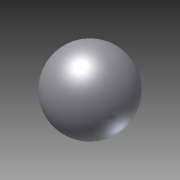
# Autodesk Inventor part: AtwoodsBall
Saved by Autodesk Inventor 2012 SP2 (Build 160219200, 219)
## iProperties
Created: 2013-07-18
Part Number: AtwoodsBall
Material: Default
Document SubType Name: Modeling
Designer: 1
Density: 1 g/cm^3
Author: 1
Autodesk Inventor part; units mm, degrees
ref_plane "YZ Plane" through (0, 0, 0) normal (1, 0, 0) x (0, 1, 0)
ref_plane "XZ Plane" through (0, 0, 0) normal (0, 1, 0) x (-1, 0, 0)
ref_plane "XY Plane" through (0, 0, 0) normal (0, 0, 1) x (1, 0, 0)
sketch "Sketch1" plane through (0, 0, 0) normal (0, 0, 1) x (1, 0, 0)
  point P0 (0, 0)
sketch "Sketch2" plane through (0, 0, 0) normal (0, 1, 0) x (-1, 0, 0)
  line L0 (-3, 0) -> (1, 0) projected
  line L1 (-3, 0) -> (1, 0) projected
  circle A0 centre (-1.1251, 15.9532) radius 15.9532
  line L2 (-1.1251, 0) -> (-1.1251, 31.9064)
  constraints: 2 end point, 2 point on circle, 1 centre point, 1 perpendicular, 1 point on line, 1 tangent
revolve "Revolution1" add sketch "Sketch2" angle 360 about axis through (1.1251, 0, 0) along (0, 0, 1)
body "Solid1"
